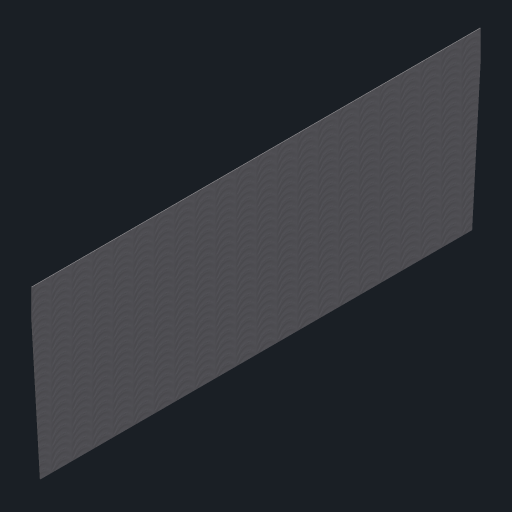
# Autodesk Inventor part: CHAPA_2
Saved by Autodesk Inventor 2024.3 (Build 283343000, 343)
## iProperties
Created: 2024-06-14
Part Number: CHAPA_2
Material: Steel, Mild, Welded
Document SubType Name: Sheet Metal
Designer: Niler
Density: 7.85 g/cm^3
Sheet Metal Rule: Default
Appearance: Weld - Steel Mild
Author: Niler
Autodesk Inventor part; units mm, degrees
ref_plane "YZ Plane" through (0, 0, 0) normal (1, 0, 0) x (0, 1, 0)
ref_plane "XZ Plane" through (0, 0, 0) normal (0, 1, 0) x (-1, 0, 0)
ref_plane "XY Plane" through (0, 0, 0) normal (0, 0, 1) x (1, 0, 0)
sketch "Sketch1" plane through (0, 0, 0) normal (1, 0, 0) x (0, 1, 0)
  line L0 (-30.5, 491.5) -> (30.5, 491.5)
  line L1 (30.5, 491.5) -> (30.5, -491.5)
  line L2 (30.5, -491.5) -> (-30.5, -491.5)
  line L3 (-30.5, -491.5) -> (-30.5, 491.5)
  line L4 (-30.5, 491.5) -> (30.5, -491.5) construction
  line L5 (30.5, 491.5) -> (-30.5, -491.5) construction
  line L6 (-30.5, 491.5) -> (-1000.3673, 433.5)
  line L7 (-1000.3673, 433.5) -> (-1000.3673, -433.5)
  line L8 (-1000.3673, -433.5) -> (-30.5, -491.5)
  line L9 (-343.5, 472.782) -> (-343.5, -472.782)
  point P0 (0, 0)
  point P1 (-1000.3673, 0)
  point P2 (-30.5, 0)
  dimension "d0" = 983
  dimension "d1" = 61
  dimension "d3" = 867
  dimension "d4" = 971.6
  dimension "d5" = 374
  measures "d0" distance of L0.end L1.end
  measures "d1" distance of L0.start L0.end
  measures "d3" distance of L6.end L7.end
  measures "d4" distance of L0.start L6.end
  measures "d5" distance between parallel lines of L9 L1
extrude "Plate1" add sketch "Sketch1" along normal blind 1.5 contours L0 L1 L2 L3 | L3 L8 L9 L6
equation "\"d6\" = Thickness"
equation "\"BendRadius\" = Thickness"
equation "\"BendReliefWidth\" = Thickness"
equation "\"BendReliefDepth\" = 0.5 * Thickness"
equation "\"CornerReliefSize\" = 4 * Thickness"
equation "\"MinimumRemnant\" = 2 * Thickness"
equation "\"TransitionRadius\" = BendRadius"
equation "\"JacobiRadiusSize\" = BendRadius"
equation "\"GapSize\" = Thickness"
equation "\"Thickness\" = 1.5"
body "Solid1"
